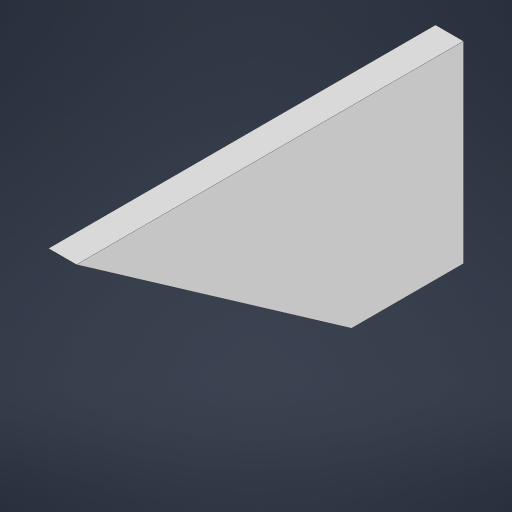
# Autodesk Inventor part: flip out sleds
Saved by Autodesk Inventor 2024 (Build 280153000, 153)
## iProperties
Created: 2024-03-28
Part Number: flip out sleds
Material: Generic
Document SubType Name: Modeling
Designer: Andrew
Density: 1 g/cm^3
Appearance: Default
Author: Andrew
Autodesk Inventor part; units mm, degrees
ref_plane "YZ Plane" through (0, 0, 0) normal (1, 0, 0) x (0, 1, 0)
ref_plane "XZ Plane" through (0, 0, 0) normal (0, 1, 0) x (-1, 0, 0)
ref_plane "XY Plane" through (0, 0, 0) normal (0, 0, 1) x (1, 0, 0)
sketch "Sketch1" plane through (0, 0, 0) normal (1, 0, 0) x (0, 1, 0)
  line L0 (0, 0) -> (0, -12.7)
  line L1 (0, 0) -> (21.8533, 31.2097)
  line L2 (21.8533, 31.2097) -> (21.8533, -12.7)
  line L3 (21.8533, -12.7) -> (0, -12.7)
  dimension "d0" = 12.7
  dimension "d1" = 38.1
  dimension "d3" = 145
  constraints: 8 end point, 2 vertical, 1 perpendicular
  measures "d0" distance of L0.start L0.end
  measures "d1" distance of L0.start L1.end
  measures "d3" angle of L0 L1
extrude "Extrusion1" add sketch "Sketch1" along normal blind 3.175
body "Solid1"
